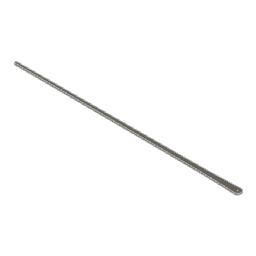
_Test Arm.1c65548c-91b3-4f5a-b04f-d94ceb853416 (Autodesk Fusion 360 design; units mm, degrees)
Autodesk Fusion 360 part; units mm, degrees
sketch "Sketch1" plane through (0, 0, 0) normal (0, 0, 1) x (1, 0, 0)
  circle A0 centre (-4.7625, 4.7625) radius 4.7625
  circle A1 centre (-4.7625, 4.7625) radius 0.5
  circle A2 centre (-304.8, 4.7625) radius 1.5875
  spline S0 degree 2 poles (-304.8, 3.175) (-39.4413, 1.9374) (-4.7625, 0) knots 0 0 0 30.006815 30.006815 30.006815 weights 1 3 1
  spline S1 degree 2 poles (-304.8, 6.35) (-40.64, 7.62) (-4.7625, 9.525) knots 0 0 0 30.006723 30.006723 30.006723 weights 1 3 1
  dimension "d3" = 1
  dimension "d4" = 3.175
  constraint concentric A0 A1
  constraint coincident A0 S0.end
  constraint coincident A2 S0.start
  constraint coincident A0 S1.end
  constraint coincident A2 S1.start
  measures "d3" diameter of A1
  measures "d4" diameter of A2
extrude "Extrude1" add sketch "Sketch1" along normal blind 2 contours A0 S0 S1 | A0 A2 S0 S1 | A2
